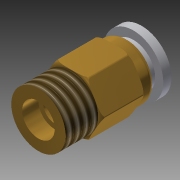
# Autodesk Inventor part: pc4_m10
Saved by Autodesk Inventor 2013 (Build 170138000, 138)
## iProperties
Created: 2015-02-20
Part Number: pc4_m10
Material: 一般
Document SubType Name: Modeling
Designer: Noa Izumi
Density: 1 g/cm^3
Author: Noa Izumi
Autodesk Inventor part; units mm, degrees
ref_plane "YZ Plane" through (0, 0, 0) normal (1, 0, 0) x (0, 1, 0)
ref_plane "XZ Plane" through (0, 0, 0) normal (0, 1, 0) x (-1, 0, 0)
ref_plane "XY Plane" through (0, 0, 0) normal (0, 0, 1) x (1, 0, 0)
sketch "草圖1" plane through (0, 0, 0) normal (0, 1, 0) x (-1, 0, 0)
  circle A0 centre (0, 0) radius 5
  dimension "d0" = 10
  constraints: 1 centre point, 1 coincident
  measures "d0" diameter of A0
extrude "擠出1" add sketch "草圖1" along normal blind 6
sketch "草圖2" plane through (0, 6, 0) normal (0, 1, 0) x (1, 0, 0)
  circle A0 centre (0, 0) radius 5 projected
  line L0 (2.8868, 5) -> (5.7735, 0)
  line L1 (5.7735, 0) -> (2.8868, -5)
  line L2 (2.8868, -5) -> (-2.8868, -5)
  line L3 (-2.8868, -5) -> (-5.7735, 0)
  line L4 (-5.7735, 0) -> (-2.8868, 5)
  line L5 (-2.8868, 5) -> (2.8868, 5)
  point P0 (0, 5)
  constraints: 12 end point, 1 coincident, 1 midpoint, 1 vertical alignment, 14 other
extrude "擠出2" add sketch "草圖2" along normal blind 8
sketch "草圖3" plane through (0, 14, 0) normal (0, 1, 0) x (1, 0, 0)
  circle A0 centre (0, 0) radius 5
  constraints: 1 centre point, 1 coincident
extrude "擠出3" add sketch "草圖3" along normal blind 2.5
fillet "圓角1" radius 1 1 edges at (-5, 16.5, 0)
sketch "草圖4" plane through (0, 16.5, 0) normal (0, 1, 0) x (1, 0, 0)
  circle A0 centre (0, 0) radius 4 projected
  circle A1 centre (0, 0) radius 4
  constraints: 1 centre point, 1 coincident, 1 concentric
extrude "擠出4" add sketch "草圖4" along normal blind 1
sketch "草圖5" plane through (0, 17.5, 0) normal (0, 1, 0) x (1, 0, 0)
  circle A0 centre (0, 0) radius 4 projected
  circle A1 centre (0, 0) radius 5.5
  dimension "d11" = 11
  constraints: 1 centre point, 1 coincident
  measures "d11" diameter of A1
extrude "擠出5" add sketch "草圖5" along normal blind 1.5 contours A0 | A1
fillet "圓角2" radius 0.25 6 edges at (5.7735, 10, 0) (2.8868, 10, 5) (2.8868, 10, -5) (-2.8868, 10, -5) (-5.7735, 10, 0) (-2.8868, 10, 5)
sketch "草圖6" plane through (0, 0, 0) normal (0, -1, 0) x (1, 0, 0)
  circle A0 centre (0, 0) radius 5 projected
  constraints: 1 coincident
hole "孔1" at (0, 0, 0) direction (0, 1, 0) diameter 6 depth 3
thread "螺紋1" size "M10x1.5" class "6g" standard "ANSI Metric M Profile" full length
sketch "草圖7" plane through (0, 19, 0) normal (0, 1, 0) x (1, 0, 0)
  circle A0 centre (0, 0) radius 5.5 projected
  constraints: 1 coincident
hole "孔2" at (0, 19, 0) direction (0, -1, 0) diameter 4 end through all
sketch "草圖8" plane through (0, 0, 0) normal (0, -1, 0) x (1, 0, 0)
  circle A0 centre (0, 0) radius 5 projected
  constraints: 1 coincident
hole "孔3" at (0, 0, 0) direction (0, 1, 0) diameter 4.2 depth 10 tip angle 118
sketch "草圖9" plane through (0, 0, 0) normal (0, 0, 1) x (1, 0, 0)
  line L0 (-5.75, 14) -> (-5, 14)
  line L1 (-5.75, 6) -> (-5, 6)
  line L2 (-5.75, 14) -> (-5.75, 13.5)
  line L3 (-5.75, 6) -> (-5.75, 6.5)
  arc A0 (-5, 14) -> (-5.75, 13.5) centre (-5, 13.1875) ccw
  arc A1 (-5.75, 6.5) -> (-5, 6) centre (-5, 6.8125) ccw
  line L4 (0, 0) -> (0, 14)
  dimension "d39" = 6
  dimension "d40" = 8
  dimension "d41" = 5
  dimension "d42" = 5
  dimension "d43" = 0.75
  dimension "d44" = 0.75
  dimension "d45" = 0.5
  dimension "d46" = 0.5
  constraints: 10 end point, 4 point on circle, 2 centre point, 2 parallel, 2 tangent, 1 collinear, 1 horizontal, 1 perpendicular
  measures "d39" distance from line of L4.start L1
  measures "d40" distance between parallel lines of L1 L0
  measures "d41" horizontal distance of L4.start L1.end
  measures "d42" horizontal distance of L4.start L0.end
  measures "d43" distance of L0.start L0.end
  measures "d44" distance of L1.start L1.end
  measures "d45" distance of L0.start L2.end
  measures "d46" distance of L1.start L3.end
revolve "迴轉1" cut sketch "草圖9" angle 360 about axis through (0, 0, 0) along (0, 1, 0)
